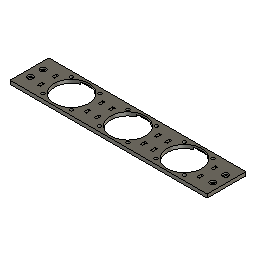
rear_fan_plate (Autodesk Fusion 360 design; units mm, degrees)
part number: 2026-08-26-07-13-35-903
Autodesk Fusion 360 part; units mm, degrees
sketch "Sketch1" plane through (0, 0, 0) normal (0, 0, 1) x (1, 0, 0)
  line L0 (-111, 0.4) -> (111, 0.4)
  line L1 (111, 0.4) -> (111, 44.05)
  line L2 (111, 44.05) -> (-111, 44.05)
  line L3 (-111, 44.05) -> (-111, 0.4)
extrude "Extrude1" add sketch "Sketch1" along normal blind 4
sketch "Sketch2" plane through (0, 0, 0) normal (0, 0, 1) x (1, 0, 0)
  circle A0 centre (-63.55, 22.225) radius 19.5
  circle A1 centre (-79.55, 6.225) radius 1.8
  circle A2 centre (-79.55, 38.225) radius 1.8
  circle A3 centre (-47.55, 6.225) radius 1.8
  circle A4 centre (-47.55, 38.225) radius 1.8
  circle A5 centre (0, 22.225) radius 19.5
  circle A6 centre (-16, 6.225) radius 1.8
  circle A7 centre (-16, 38.225) radius 1.8
  circle A8 centre (16, 6.225) radius 1.8
  circle A9 centre (16, 38.225) radius 1.8
  circle A10 centre (63.55, 22.225) radius 19.5
  circle A11 centre (47.55, 6.225) radius 1.8
  circle A12 centre (47.55, 38.225) radius 1.8
  circle A13 centre (79.55, 6.225) radius 1.8
  circle A14 centre (79.55, 38.225) radius 1.8
  circle A15 centre (-102.82, 15) radius 1.7
  circle A16 centre (-102.82, 29.45) radius 1.7
  circle A17 centre (102.82, 15) radius 1.7
  circle A18 centre (102.82, 29.45) radius 1.7
extrude "Extrude2" cut sketch "Sketch2" along normal blind 4
sketch "Sketch3" plane through (0, 0, 0) normal (0, 0, 1) x (1, 0, 0)
  line L0 (-90.8, 11.5) -> (-88.3, 11.5)
  line L1 (-88.3, 11.5) -> (-88.3, 16.5)
  line L2 (-88.3, 16.5) -> (-90.8, 16.5)
  line L3 (-90.8, 16.5) -> (-90.8, 11.5)
  line L4 (-90.8, 27.5) -> (-88.3, 27.5)
  line L5 (-88.3, 27.5) -> (-88.3, 32.5)
  line L6 (-88.3, 32.5) -> (-90.8, 32.5)
  line L7 (-90.8, 32.5) -> (-90.8, 27.5)
  line L8 (-38.8, 11.5) -> (-36.3, 11.5)
  line L9 (-36.3, 11.5) -> (-36.3, 16.5)
  line L10 (-36.3, 16.5) -> (-38.8, 16.5)
  line L11 (-38.8, 16.5) -> (-38.8, 11.5)
  line L12 (-38.8, 27.5) -> (-36.3, 27.5)
  line L13 (-36.3, 27.5) -> (-36.3, 32.5)
  line L14 (-36.3, 32.5) -> (-38.8, 32.5)
  line L15 (-38.8, 32.5) -> (-38.8, 27.5)
  line L16 (-27.25, 11.5) -> (-24.75, 11.5)
  line L17 (-24.75, 11.5) -> (-24.75, 16.5)
  line L18 (-24.75, 16.5) -> (-27.25, 16.5)
  line L19 (-27.25, 16.5) -> (-27.25, 11.5)
  line L20 (-27.25, 27.5) -> (-24.75, 27.5)
  line L21 (-24.75, 27.5) -> (-24.75, 32.5)
  line L22 (-24.75, 32.5) -> (-27.25, 32.5)
  line L23 (-27.25, 32.5) -> (-27.25, 27.5)
  line L24 (24.75, 11.5) -> (27.25, 11.5)
  line L25 (27.25, 11.5) -> (27.25, 16.5)
  line L26 (27.25, 16.5) -> (24.75, 16.5)
  line L27 (24.75, 16.5) -> (24.75, 11.5)
  line L28 (24.75, 27.5) -> (27.25, 27.5)
  line L29 (27.25, 27.5) -> (27.25, 32.5)
  line L30 (27.25, 32.5) -> (24.75, 32.5)
  line L31 (24.75, 32.5) -> (24.75, 27.5)
  line L32 (36.3, 11.5) -> (38.8, 11.5)
  line L33 (38.8, 11.5) -> (38.8, 16.5)
  line L34 (38.8, 16.5) -> (36.3, 16.5)
  line L35 (36.3, 16.5) -> (36.3, 11.5)
  line L36 (36.3, 27.5) -> (38.8, 27.5)
  line L37 (38.8, 27.5) -> (38.8, 32.5)
  line L38 (38.8, 32.5) -> (36.3, 32.5)
  line L39 (36.3, 32.5) -> (36.3, 27.5)
  line L40 (88.3, 11.5) -> (90.8, 11.5)
  line L41 (90.8, 11.5) -> (90.8, 16.5)
  line L42 (90.8, 16.5) -> (88.3, 16.5)
  line L43 (88.3, 16.5) -> (88.3, 11.5)
  line L44 (88.3, 27.5) -> (90.8, 27.5)
  line L45 (90.8, 27.5) -> (90.8, 32.5)
  line L46 (90.8, 32.5) -> (88.3, 32.5)
  line L47 (88.3, 32.5) -> (88.3, 27.5)
extrude "Extrude3" cut sketch "Sketch3" along normal blind 4
ref_plane "WorkPlane1" through (0, 0, 4) normal (0, 0, 1) x (1, 0, 0)
sketch "Sketch4" plane through (0, 0, 4) normal (0, 0, 1) x (1, 0, 0)
  circle A0 centre (-102.82, 15) radius 3.25
  circle A1 centre (-102.82, 29.45) radius 3.25
  circle A2 centre (102.82, 15) radius 3.25
  circle A3 centre (102.82, 29.45) radius 3.25
extrude "Extrude4" cut sketch "Sketch4" against normal blind 2
sketch "Sketch5" plane through (0, 0, 0) normal (0, 0, 1) x (1, 0, 0)
  line L0 (-97.6, 2) -> (97.6, 2)
  line L1 (97.6, 2) -> (97.6, 4.4)
  line L2 (97.6, 4.4) -> (-97.6, 4.4)
  line L3 (-97.6, 4.4) -> (-97.6, 2)
  line L4 (-97.6, 40.05) -> (97.6, 40.05)
  line L5 (97.6, 40.05) -> (97.6, 42.45)
  line L6 (97.6, 42.45) -> (-97.6, 42.45)
  line L7 (-97.6, 42.45) -> (-97.6, 40.05)
extrude "Extrude5" cut sketch "Sketch5" along normal blind 2
named bodies: "Rear Fan Plate"
